Autodesk Inventor part; units mm, degrees
(part 2 of 2)
  spline S177 degree 3 poles (4.8169, 39.172) (4.6782, 38.9898) (4.5503, 38.7988) (4.3217, 38.3936) (4.2159, 38.1797) (4.0576, 37.7838) (3.993, 37.6061) (3.9199, 37.304) (3.8938, 37.1823) (3.8938, 37.0599) knots 0 0 0 0 0.294801 0.294801 0.599477 0.599477 0.842158 0.842158 1 1 1 1
  spline S178 degree 3 poles (22.2511, 37.2023) (22.2293, 37.2635) (22.2074, 37.3246) (22.1616, 37.453) (22.1204, 37.5159) (22.0066, 37.5961) (21.9396, 37.6167) (21.8732, 37.6167) knots 0 0 0 0 0.319996 0.319996 0.672558 0.672558 1 1 1 1
  spline S179 degree 2 poles (22.2511, 37.2023) (22.2677, 37.1877) (22.3899, 37.1012) (22.5179, 37.1012) knots 0.820738 0.820738 0.820738 1 2 2 2
  spline S180 degree 2 poles (22.5179, 37.1012) (22.6319, 37.1012) (22.8367, 37.2176) (22.9112, 37.3246) knots 0 0 0 1 2 2 2
  spline S181 degree 2 poles (22.9112, 37.3246) (23.0446, 37.5226) (23.0786, 38.0049) knots 0 0 0 0.924384 0.924384 0.924384
  spline S182 degree 3 poles (22.4225, 37.7192) (22.5545, 37.7192) (22.6891, 37.7457) (22.91, 37.8523) (23.001, 37.9228) (23.0786, 38.0049) knots 0 0 0 0 0.540011 0.540011 1 1 1 1
  spline S183 degree 3 poles (21.4881, 38.7257) (21.4881, 38.5944) (21.5102, 38.4625) (21.5981, 38.2196) (21.6635, 38.1074) (21.8327, 37.9218) (21.9363, 37.8474) (22.1658, 37.7449) (22.2953, 37.7192) (22.4225, 37.7192) knots 0 0 0 0 0.25832 0.25832 0.506669 0.506669 0.749947 0.749947 1 1 1 1
  spline S184 degree 3 poles (22.5505, 39.7812) (22.4044, 39.7812) (22.2546, 39.7563) (21.9944, 39.649) (21.8771, 39.5727) (21.687, 39.3809) (21.6123, 39.2629) (21.5132, 39.007) (21.4881, 38.865) (21.4881, 38.7257) knots 0 0 0 0 0.263162 0.263162 0.506642 0.506642 0.74915 0.74915 1 1 1 1
  spline S185 degree 3 poles (23.692, 38.2882) (23.692, 38.5011) (23.6719, 38.7154) (23.5699, 39.09) (23.5008, 39.2539) (23.2994, 39.5163) (23.1745, 39.617) (22.8834, 39.7517) (22.7151, 39.7812) (22.5505, 39.7812) knots 0 0 0 0 0.301479 0.301479 0.547676 0.547676 0.76686 0.76686 1 1 1 1
  spline S186 degree 3 poles (22.5016, 36.6672) (22.6714, 36.6672) (22.8436, 36.6978) (23.1467, 36.8392) (23.2768, 36.9507) (23.4893, 37.2339) (23.5642, 37.4125) (23.6719, 37.8193) (23.692, 38.0562) (23.692, 38.2882) knots 0 0 0 0 0.225089 0.225089 0.443165 0.443165 0.692425 0.692425 1 1 1 1
  spline S187 degree 3 poles (21.6021, 37.3479) (21.6021, 37.2366) (21.6487, 37.1295) (21.7902, 36.9229) (21.9024, 36.8362) (22.1707, 36.6973) (22.3382, 36.6672) (22.5016, 36.6672) knots 0 0 0 0 0.270338 0.270338 0.603095 0.603095 1 1 1 1
  spline S188 degree 3 poles (21.8732, 37.6167) (21.832, 37.6167) (21.7593, 37.6021) (21.6999, 37.5572) (21.6517, 37.5063) (21.6132, 37.447) (21.6021, 37.3773) (21.6021, 37.3479) knots 0 0 0 0 0.292922 0.512613 0.512613 0.79112 1 1 1 1
  spline S189 degree 3 poles (30.4375, 39.79) (30.4036, 39.79) (30.3434, 39.7855) (30.2892, 39.7567) (30.2556, 39.7208) (30.2301, 39.6882) (30.1801, 39.622) (30.1454, 39.5737) (30.0482, 39.4385) (29.964, 39.3461) (29.8067, 39.2089) (29.6828, 39.1259) (29.5498, 39.058) (29.4923, 39.0312) knots 0 0 0 0 0.081756 0.143072 0.143072 0.200115 0.242897 0.342722 0.342722 0.642421 0.642421 0.846752 1 1 1 1
  spline S190 degree 3 poles (30.7225, 39.4304) (30.7225, 39.5212) (30.704, 39.6157) (30.6197, 39.7246) (30.5541, 39.7767) (30.472, 39.79) (30.4375, 39.79) knots 0 0 0 0 0.529945 0.529945 0.798548 1 1 1 1
  line L67 (30.7225, 37.1263) -> (30.7225, 39.4304)
  spline S191 degree 3 poles (30.3979, 36.6714) (30.458, 36.6714) (30.5831, 36.7004) (30.6846, 36.8431) (30.7171, 36.9901) (30.7225, 37.0812) (30.7225, 37.1263) knots 0 0 0 0 0.285714 0.571429 0.785714 1 1 1 1
  spline S192 degree 3 poles (30.0756, 37.0472) (30.0756, 36.9489) (30.0968, 36.8439) (30.1964, 36.7333) (30.2718, 36.6832) (30.3606, 36.6714) (30.3979, 36.6714) knots 0 0 0 0 0.52997 0.52997 0.798558 1 1 1 1
  line L68 (30.0756, 38.7782) -> (30.0756, 37.0472)
  spline S193 degree 3 poles (29.4367, 38.4355) (29.4764, 38.4355) (29.5541, 38.4558) (29.6987, 38.5229) (29.8728, 38.6311) (30.0071, 38.7271) (30.0756, 38.7782) knots 0 0 0 0 0.162539 0.325077 0.650155 1 1 1 1
  spline S194 degree 3 poles (29.1726, 38.709) (29.1726, 38.6688) (29.1882, 38.5983) (29.2307, 38.5401) (29.2794, 38.4897) (29.337, 38.4482) (29.4071, 38.4355) (29.4367, 38.4355) knots 0 0 0 0 0.288261 0.504456 0.504456 0.787624 1 1 1 1
  spline S195 degree 3 poles (29.4923, 39.0312) (29.4457, 39.0092) (29.3647, 38.9693) (29.287, 38.9235) (29.2317, 38.8813) (29.1847, 38.8236) (29.1726, 38.75) (29.1726, 38.709) knots 0 0 0 0 0.317971 0.55645 0.55645 0.746543 1 1 1 1
  spline S196 degree 3 poles (39.388, 39.7748) (39.3541, 39.7748) (39.2939, 39.7702) (39.2397, 39.7415) (39.2101, 39.7099) (39.1842, 39.6777) (39.1341, 39.6115) (39.0958, 39.5585) (38.9987, 39.4233) (38.9145, 39.3308) (38.7572, 39.1936) (38.6333, 39.1107) (38.5003, 39.0428) (38.4428, 39.016) knots 0 0 0 0 0.081756 0.143072 0.143072 0.185854 0.242897 0.342722 0.342722 0.642421 0.642421 0.846752 1 1 1 1
  spline S197 degree 3 poles (39.673, 39.4152) (39.673, 39.506) (39.6545, 39.6005) (39.5773, 39.7002) (39.516, 39.7561) (39.434, 39.7748) (39.388, 39.7748) knots 0 0 0 0 0.529945 0.529945 0.731397 1 1 1 1
  line L69 (39.673, 37.1111) -> (39.673, 39.4152)
  spline S198 degree 3 poles (39.3484, 36.6561) (39.4085, 36.6561) (39.5335, 36.6852) (39.6351, 36.8278) (39.6676, 36.9748) (39.673, 37.066) (39.673, 37.1111) knots 0 0 0 0 0.285714 0.571429 0.785714 1 1 1 1
  spline S199 degree 3 poles (39.0261, 37.032) (39.0261, 36.9337) (39.0473, 36.8286) (39.1469, 36.7181) (39.2223, 36.668) (39.311, 36.6561) (39.3484, 36.6561) knots 0 0 0 0 0.52997 0.52997 0.798558 1 1 1 1
  line L70 (39.0261, 38.763) -> (39.0261, 37.032)
  spline S200 degree 3 poles (38.3872, 38.4203) (38.4269, 38.4203) (38.5046, 38.4406) (38.6492, 38.5077) (38.8233, 38.6159) (38.9576, 38.7119) (39.0261, 38.763) knots 0 0 0 0 0.162539 0.325077 0.650155 1 1 1 1
  spline S201 degree 3 poles (38.1231, 38.6937) (38.1231, 38.6535) (38.1387, 38.583) (38.1812, 38.5249) (38.2229, 38.4817) (38.278, 38.4376) (38.3477, 38.4203) (38.3872, 38.4203) knots 0 0 0 0 0.288261 0.504456 0.504456 0.716832 1 1 1 1
  spline S202 degree 3 poles (38.4428, 39.016) (38.3962, 38.994) (38.3152, 38.9541) (38.2375, 38.9082) (38.1822, 38.866) (38.1352, 38.8084) (38.1231, 38.7348) (38.1231, 38.6937) knots 0 0 0 0 0.317971 0.55645 0.55645 0.746543 1 1 1 1
  spline S203 degree 3 poles (48.4842, 39.7369) (48.4503, 39.7369) (48.3901, 39.7324) (48.3359, 39.7036) (48.3023, 39.6677) (48.2768, 39.6351) (48.2268, 39.569) (48.1921, 39.5207) (48.0949, 39.3854) (48.0107, 39.293) (47.8534, 39.1558) (47.7295, 39.0729) (47.5965, 39.005) (47.539, 38.9781) knots 0 0 0 0 0.081756 0.143072 0.143072 0.200115 0.242897 0.342722 0.342722 0.642421 0.642421 0.846752 1 1 1 1
  spline S204 degree 3 poles (48.7692, 39.3774) (48.7692, 39.4682) (48.7507, 39.5627) (48.6664, 39.6716) (48.6008, 39.7236) (48.5187, 39.7369) (48.4842, 39.7369) knots 0 0 0 0 0.529945 0.529945 0.798548 1 1 1 1
  line L71 (48.7692, 37.0733) -> (48.7692, 39.3774)
  spline S205 degree 3 poles (48.4446, 36.6183) (48.4897, 36.6183) (48.582, 36.6325) (48.7035, 36.7317) (48.7612, 36.8925) (48.7692, 37.0132) (48.7692, 37.0733) knots 0 0 0 0 0.214286 0.428571 0.714286 1 1 1 1
  spline S206 degree 3 poles (48.1223, 36.9942) (48.1223, 36.8959) (48.1435, 36.7908) (48.2348, 36.6896) (48.3059, 36.6349) (48.3948, 36.6183) (48.4446, 36.6183) knots 0 0 0 0 0.52997 0.52997 0.731411 1 1 1 1
  line L72 (48.1223, 38.7252) -> (48.1223, 36.9942)
  spline S207 degree 3 poles (47.4834, 38.3825) (47.5231, 38.3825) (47.6008, 38.4028) (47.7454, 38.4699) (47.9195, 38.578) (48.0538, 38.6741) (48.1223, 38.7252) knots 0 0 0 0 0.162539 0.325077 0.650155 1 1 1 1
  spline S208 degree 3 poles (47.2193, 38.6559) (47.2193, 38.6258) (47.2306, 38.5551) (47.2704, 38.4943) (47.3261, 38.4367) (47.3837, 38.3952) (47.4538, 38.3825) (47.4834, 38.3825) knots 0 0 0 0 0.216195 0.504456 0.504456 0.787624 1 1 1 1
  spline S209 degree 3 poles (47.539, 38.9781) (47.4924, 38.9562) (47.4114, 38.9162) (47.3337, 38.8704) (47.2784, 38.8282) (47.2314, 38.7706) (47.2193, 38.6969) (47.2193, 38.6559) knots 0 0 0 0 0.317971 0.55645 0.55645 0.746543 1 1 1 1
  spline S210 degree 3 poles (-13.2698, 38.7932) (-13.2836, 38.7932) (-13.2975, 38.7929) (-13.3252, 38.7915) (-13.3392, 38.7905) (-13.3602, 38.7885) (-13.3672, 38.7877) (-13.3884, 38.7852) (-13.4025, 38.7831) (-13.4238, 38.7796) (-13.4309, 38.7784) (-13.4524, 38.7743) (-13.4667, 38.7713) (-13.4882, 38.7663) (-13.4954, 38.7646) (-13.5172, 38.7591) (-13.5317, 38.7551) (-13.5534, 38.7486) (-13.5607, 38.7464) (-13.5827, 38.7394) (-13.5974, 38.7344) (-13.6194, 38.7266) (-13.6268, 38.7239) (-13.6491, 38.7154) (-13.664, 38.7095) (-13.6863, 38.7002) (-13.6937, 38.697) (-13.7019, 38.6935) (-13.7026, 38.6932) (-13.7033, 38.6929) knots 0 0 0 0 0.092703 0.092703 0.186345 0.186345 0.233583 0.233583 0.329041 0.329041 0.377326 0.377326 0.475187 0.475187 0.52484 0.52484 0.625741 0.625741 0.676923 0.676923 0.780779 0.780779 0.833489 0.833489 0.940578 0.940578 0.995003 0.995003 1 1 1 1
  spline S211 degree 3 poles (-12.2735, 37.7713) (-12.2735, 37.8182) (-12.2763, 37.8652) (-12.2863, 37.946) (-12.2922, 37.9799) (-12.3023, 38.0245) (-12.305, 38.0356) (-12.3136, 38.0685) (-12.3201, 38.0902) (-12.3308, 38.1223) (-12.3346, 38.133) (-12.3464, 38.1646) (-12.355, 38.1854) (-12.3688, 38.2159) (-12.3735, 38.226) (-12.3879, 38.2556) (-12.3981, 38.275) (-12.4144, 38.3036) (-12.4199, 38.313) (-12.4425, 38.3499) (-12.4608, 38.3768) (-12.4933, 38.4198) (-12.5069, 38.4365) (-12.5493, 38.4854) (-12.5795, 38.5159) (-12.6276, 38.5585) (-12.6439, 38.5722) (-12.6943, 38.6114) (-12.7297, 38.6354) (-12.7848, 38.6679) (-12.8036, 38.6782) (-12.8616, 38.7075) (-12.9014, 38.7248) (-12.9631, 38.7465) (-12.9841, 38.7529) (-13.0477, 38.7703) (-13.0911, 38.7789) (-13.1797, 38.7905) (-13.225, 38.7932) (-13.2698, 38.7932) knots 0 0 0 0 0.088924 0.088924 0.154115 0.154115 0.175635 0.175635 0.218439 0.218439 0.239813 0.239813 0.282415 0.282415 0.303307 0.303307 0.344643 0.344643 0.365106 0.365106 0.426005 0.426005 0.466506 0.466506 0.547908 0.547908 0.588064 0.588064 0.668181 0.668181 0.708462 0.708462 0.790774 0.790774 0.832059 0.832059 0.914902 0.914902 1 1 1 1
  spline S212 degree 3 poles (-13.4188, 36.6493) (-13.3638, 36.6493) (-13.3086, 36.6523) (-13.2013, 36.6647) (-13.1493, 36.6739) (-13.0729, 36.6928) (-13.0481, 36.6998) (-12.9871, 36.7193) (-12.9513, 36.7328) (-12.9048, 36.7533) (-12.8933, 36.7586) (-12.8592, 36.775) (-12.8369, 36.7868) (-12.8041, 36.8056) (-12.7934, 36.812) (-12.7514, 36.8379) (-12.7209, 36.8587) (-12.6724, 36.8958) (-12.6537, 36.9111) (-12.5995, 36.9588) (-12.5659, 36.9927) (-12.5191, 37.0474) (-12.5042, 37.0661) (-12.4685, 37.1143) (-12.4486, 37.1445) (-12.4241, 37.186) (-12.4182, 37.1966) (-12.4008, 37.2285) (-12.3899, 37.2501) (-12.3747, 37.2829) (-12.3698, 37.2939) (-12.351, 37.3382) (-12.3385, 37.3721) (-12.3204, 37.4297) (-12.3139, 37.453) (-12.2965, 37.524) (-12.2878, 37.5723) (-12.2763, 37.671) (-12.2735, 37.7213) (-12.2735, 37.7713) knots 0 0 0 0 0.092276 0.092276 0.180807 0.180807 0.223969 0.223969 0.287955 0.287955 0.309124 0.309124 0.351194 0.351194 0.372002 0.372002 0.43328 0.43328 0.47363 0.47363 0.553801 0.553801 0.593615 0.593615 0.653557 0.653557 0.673705 0.673705 0.713981 0.713981 0.734138 0.734138 0.794581 0.794581 0.834843 0.834843 0.916161 0.916161 1 1 1 1
  spline S213 degree 3 poles (-14.4849, 37.4571) (-14.4849, 37.4309) (-14.4824, 37.4046) (-14.4733, 37.351) (-14.4665, 37.3237) (-14.4537, 37.2829) (-14.4488, 37.2689) (-14.4352, 37.2331) (-14.426, 37.2115) (-14.4126, 37.1829) (-14.4091, 37.1755) (-14.3999, 37.1569) (-14.3941, 37.1458) (-14.3861, 37.1308) (-14.3841, 37.1269) (-14.3776, 37.1151) (-14.373, 37.1072) (-14.3659, 37.0954) (-14.3635, 37.0914) (-14.3535, 37.0757) (-14.3457, 37.0641) (-14.332, 37.0451) (-14.3263, 37.0376) (-14.3087, 37.015) (-14.2963, 37.0004) (-14.2768, 36.9789) (-14.2701, 36.9718) (-14.2421, 36.9432) (-14.2199, 36.9227) (-14.1809, 36.89) (-14.1645, 36.8771) (-14.1258, 36.8484) (-14.1034, 36.833) (-14.0759, 36.8153) (-14.0711, 36.8123) (-14.0568, 36.8033) (-14.0471, 36.7974) (-14.0322, 36.7887) (-14.0271, 36.7857) (-14.0062, 36.774) (-13.9901, 36.7656) (-13.9629, 36.7525) (-13.9518, 36.7475) (-13.9061, 36.7277) (-13.8707, 36.715) (-13.8099, 36.6966) (-13.7847, 36.69) (-13.7059, 36.6721) (-13.6514, 36.6636) (-13.5374, 36.6519) (-13.4778, 36.6493) (-13.4188, 36.6493) knots 0 0 0 0 0.05342 0.05342 0.110323 0.110323 0.140525 0.140525 0.188212 0.188212 0.204851 0.204851 0.230452 0.230452 0.239326 0.239326 0.257866 0.257866 0.26723 0.26723 0.295467 0.295467 0.314492 0.314492 0.353157 0.353157 0.372878 0.372878 0.434045 0.434045 0.476554 0.476554 0.531612 0.531612 0.542912 0.542912 0.565933 0.565933 0.577878 0.577878 0.614515 0.614515 0.639286 0.639286 0.715798 0.715798 0.768641 0.768641 0.879679 0.879679 1 1 1 1
  spline S214 degree 3 poles (-14.1845, 37.7482) (-14.198, 37.7482) (-14.2116, 37.7474) (-14.2384, 37.744) (-14.2515, 37.7414) (-14.2709, 37.7361) (-14.2773, 37.7342) (-14.2962, 37.7276) (-14.3084, 37.7223) (-14.3261, 37.7131) (-14.3319, 37.7098) (-14.3461, 37.701) (-14.3543, 37.6953) (-14.365, 37.6871) (-14.3676, 37.685) (-14.3754, 37.6786) (-14.3804, 37.6741) (-14.3878, 37.6672) (-14.3902, 37.6648) (-14.3973, 37.6576) (-14.4019, 37.6527) (-14.4084, 37.6454) (-14.4105, 37.643) (-14.4166, 37.6358) (-14.4206, 37.6309) (-14.4264, 37.6233) (-14.4282, 37.6208) (-14.4355, 37.6107) (-14.4407, 37.603) (-14.4486, 37.5897) (-14.4516, 37.5844) (-14.46, 37.5682) (-14.465, 37.5571) (-14.4712, 37.54) (-14.4731, 37.5342) (-14.4781, 37.5169) (-14.4807, 37.505) (-14.4841, 37.4812) (-14.4849, 37.4691) (-14.4849, 37.4571) knots 0 0 0 0 0.088245 0.088245 0.175465 0.175465 0.21879 0.21879 0.305396 0.305396 0.348669 0.348669 0.41348 0.41348 0.435158 0.435158 0.478569 0.478569 0.5006 0.5006 0.543973 0.543973 0.564583 0.564583 0.605632 0.605632 0.625924 0.625924 0.68612 0.68612 0.725881 0.725881 0.804934 0.804934 0.844081 0.844081 0.921896 0.921896 1 1 1 1
  spline S215 degree 3 poles (-13.8701, 37.5135) (-13.88, 37.5366) (-13.8912, 37.5593) (-13.9133, 37.5962) (-13.9234, 37.611) (-13.9381, 37.6297) (-13.9418, 37.6342) (-13.9531, 37.6473) (-13.961, 37.6557) (-13.9734, 37.6675) (-13.9777, 37.6713) (-13.9905, 37.6823) (-13.9995, 37.6892) (-14.0135, 37.6988) (-14.0182, 37.7019) (-14.0326, 37.7106) (-14.0425, 37.7158) (-14.0578, 37.7228) (-14.0629, 37.725) (-14.0785, 37.7311) (-14.0892, 37.7346) (-14.1055, 37.739) (-14.111, 37.7403) (-14.1276, 37.7437) (-14.1388, 37.7454) (-14.1616, 37.7477) (-14.1731, 37.7482) (-14.1845, 37.7482) knots 0 0 0 0 0.180992 0.180992 0.309668 0.309668 0.351501 0.351501 0.434189 0.434189 0.475017 0.475017 0.555697 0.555697 0.595796 0.595796 0.676019 0.676019 0.716301 0.716301 0.796698 0.796698 0.836889 0.836889 0.917728 0.917728 1 1 1 1
  ellipse E0 centre (-13.6776, 37.5949) end of major axis (-13.766, 37.7956) minor radius 0.2091 (-13.8701, 37.5135) -> (-13.8672, 37.5069) ccw
  spline S216 degree 3 poles (-13.4095, 37.1734) (-13.4255, 37.1734) (-13.4416, 37.1741) (-13.4732, 37.1773) (-13.4887, 37.1797) (-13.5114, 37.1844) (-13.5189, 37.1862) (-13.5411, 37.1921) (-13.5556, 37.1968) (-13.5769, 37.205) (-13.5839, 37.2079) (-13.605, 37.2174) (-13.6188, 37.2245) (-13.6391, 37.2363) (-13.6458, 37.2405) (-13.6661, 37.2537) (-13.6792, 37.2634) (-13.6984, 37.2788) (-13.7047, 37.2841) (-13.7235, 37.3007) (-13.7355, 37.3123) (-13.7528, 37.3307) (-13.7586, 37.3371) (-13.7755, 37.3568) (-13.7864, 37.3706) (-13.8019, 37.3921) (-13.807, 37.3995) (-13.8222, 37.4225) (-13.8318, 37.4385) (-13.8503, 37.4719) (-13.8591, 37.4893) (-13.8672, 37.5069) knots 0 0 0 0 0.080666 0.080666 0.158277 0.158277 0.196485 0.196485 0.272757 0.272757 0.311136 0.311136 0.388673 0.388673 0.428088 0.428088 0.509412 0.509412 0.550797 0.550797 0.634906 0.634906 0.677634 0.677634 0.764932 0.764932 0.809746 0.809746 0.902371 0.902371 1 1 1 1
  spline S217 degree 3 poles (-12.9651, 37.7248) (-12.9651, 37.6979) (-12.9663, 37.6709) (-12.9711, 37.6187) (-12.9746, 37.5935) (-12.9819, 37.5567) (-12.9845, 37.5448) (-12.9933, 37.51) (-13.0004, 37.4874) (-13.0128, 37.4544) (-13.0172, 37.4438) (-13.0309, 37.4131) (-13.041, 37.3935) (-13.0581, 37.3655) (-13.0639, 37.3566) (-13.0818, 37.3312) (-13.0948, 37.3153) (-13.1157, 37.293) (-13.1229, 37.286) (-13.1451, 37.2655) (-13.161, 37.2529) (-13.186, 37.2359) (-13.1945, 37.2305) (-13.2203, 37.2156) (-13.2382, 37.2071) (-13.2658, 37.1966) (-13.2752, 37.1934) (-13.3043, 37.1848) (-13.3243, 37.1805) (-13.3661, 37.1747) (-13.3879, 37.1734) (-13.4095, 37.1734) knots 0 0 0 0 0.101982 0.101982 0.198078 0.198078 0.244289 0.244289 0.333652 0.333652 0.37732 0.37732 0.460741 0.460741 0.500448 0.500448 0.577702 0.577702 0.615856 0.615856 0.691855 0.691855 0.729606 0.729606 0.804116 0.804116 0.841589 0.841589 0.918244 0.918244 1 1 1 1
  spline S218 degree 3 poles (-13.4025, 38.2576) (-13.3823, 38.2576) (-13.362, 38.2564) (-13.3228, 38.2515) (-13.3039, 38.2479) (-13.2763, 38.2406) (-13.2673, 38.2379) (-13.2407, 38.2289) (-13.2235, 38.2217) (-13.1985, 38.2091) (-13.1902, 38.2047) (-13.1663, 38.1905) (-13.1511, 38.1798) (-13.1297, 38.162) (-13.1227, 38.1558) (-13.1019, 38.1357) (-13.089, 38.1212) (-13.0708, 38.0976) (-13.0649, 38.0892) (-13.0471, 38.0626) (-13.0362, 38.0436) (-13.0214, 38.0139) (-13.0167, 38.0036) (-13.0032, 37.9713) (-12.9957, 37.949) (-12.9862, 37.9141) (-12.9834, 37.902) (-12.9754, 37.8639) (-12.9716, 37.8376) (-12.9663, 37.7824) (-12.9651, 37.7534) (-12.9651, 37.7248) knots 0 0 0 0 0.07838 0.07838 0.152885 0.152885 0.18919 0.18919 0.261457 0.261457 0.297443 0.297443 0.36848 0.36848 0.404641 0.404641 0.480054 0.480054 0.519572 0.519572 0.603431 0.603431 0.647357 0.647357 0.738828 0.738828 0.786932 0.786932 0.888762 0.888762 1 1 1 1
  spline S219 degree 3 poles (-14.0937, 37.962) (-14.0827, 37.962) (-14.0717, 37.9628) (-14.0497, 37.9658) (-14.0387, 37.968) (-14.0223, 37.9722) (-14.0168, 37.9738) (-13.9942, 37.9809) (-13.9777, 37.9874) (-13.95, 38.0001) (-13.9387, 38.0058) (-13.9098, 38.0216) (-13.8924, 38.0323) (-13.8694, 38.0474) (-13.8634, 38.0515) (-13.8483, 38.062) (-13.8392, 38.0685) (-13.8272, 38.0775) (-13.8241, 38.0797) (-13.8154, 38.0863) (-13.8097, 38.0906) (-13.8013, 38.097) (-13.7985, 38.099) (-13.7878, 38.1071) (-13.7797, 38.1131) (-13.7666, 38.1228) (-13.7615, 38.1265) (-13.7467, 38.1373) (-13.7369, 38.1443) (-13.7226, 38.1545) (-13.718, 38.1577) (-13.7048, 38.167) (-13.6962, 38.1729) (-13.6835, 38.1816) (-13.6794, 38.1843) (-13.6679, 38.1919) (-13.6604, 38.1969) (-13.6494, 38.2039) (-13.6459, 38.2061) (-13.6376, 38.2112) (-13.6328, 38.2142) (-13.6265, 38.218) (-13.625, 38.2189) (-13.6213, 38.221) (-13.6191, 38.2223) (-13.6163, 38.2239) (-13.6156, 38.2242) (-13.614, 38.2251) (-13.613, 38.2257) (-13.6115, 38.2265) (-13.6109, 38.2268) (-13.6076, 38.2284) (-13.6047, 38.2298) (-13.5991, 38.2321) (-13.5964, 38.2332) (-13.5839, 38.2378) (-13.5737, 38.2406) (-13.5553, 38.245) (-13.5469, 38.2466) (-13.5185, 38.2515) (-13.4981, 38.2537) (-13.4525, 38.2569) (-13.4273, 38.2576) (-13.4025, 38.2576) knots 0 0 0 0 0.042878 0.042878 0.086235 0.086235 0.108331 0.108331 0.177769 0.177769 0.226997 0.226997 0.306227 0.306227 0.334276 0.334276 0.378117 0.378117 0.392867 0.392867 0.420693 0.420693 0.434144 0.434144 0.473134 0.473134 0.49792 0.49792 0.54464 0.54464 0.56656 0.56656 0.607505 0.607505 0.62651 0.62651 0.661461 0.661461 0.677346 0.677346 0.699322 0.699322 0.706098 0.706098 0.715907 0.715907 0.718762 0.718762 0.723223 0.723223 0.725491 0.725491 0.737857 0.737857 0.749199 0.749199 0.790187 0.790187 0.823398 0.823398 0.902976 0.902976 1 1 1 1
  spline S220 degree 3 poles (-14.4151, 38.269) (-14.4151, 38.2676) (-14.4151, 38.2661) (-14.4151, 38.2514) (-14.4141, 38.2381) (-14.4103, 38.2117) (-14.4074, 38.1987) (-14.4016, 38.1797) (-14.3994, 38.1734) (-14.3922, 38.1547) (-14.3864, 38.1427) (-14.3766, 38.1253) (-14.3731, 38.1195) (-14.3619, 38.1026) (-14.3537, 38.0918) (-14.3403, 38.0763) (-14.3356, 38.0712) (-14.321, 38.0562) (-14.3108, 38.0467) (-14.2946, 38.0333) (-14.2891, 38.029) (-14.2725, 38.0168) (-14.261, 38.0093) (-14.2432, 37.9992) (-14.2372, 37.9961) (-14.219, 37.9872) (-14.2065, 37.9821) (-14.1872, 37.9757) (-14.1807, 37.9738) (-14.1611, 37.9687) (-14.1478, 37.9662) (-14.1209, 37.9628) (-14.1072, 37.962) (-14.0937, 37.962) knots 0 0 0 0 0.008781 0.008781 0.090256 0.090256 0.170943 0.170943 0.211408 0.211408 0.29299 0.29299 0.333922 0.333922 0.416357 0.416357 0.458304 0.458304 0.544271 0.544271 0.586412 0.586412 0.669662 0.669662 0.711114 0.711114 0.793793 0.793793 0.834866 0.834866 0.916953 0.916953 1 1 1 1
  line L73 (-14.2222, 39.3838) -> (-14.4151, 38.269)
  spline S221 degree 3 poles (-13.8005, 39.7661) (-13.8204, 39.7661) (-13.8405, 39.7653) (-13.8792, 39.7622) (-13.8979, 39.7598) (-13.9253, 39.7548) (-13.9341, 39.7529) (-13.9598, 39.7467) (-13.9765, 39.7416) (-14.0007, 39.7323) (-14.0085, 39.729) (-14.0275, 39.72) (-14.0385, 39.714) (-14.0526, 39.7052) (-14.0561, 39.7029) (-14.0663, 39.6959) (-14.0728, 39.6909) (-14.0823, 39.6831) (-14.0855, 39.6804) (-14.0974, 39.6696) (-14.1058, 39.6609) (-14.1188, 39.6457) (-14.1237, 39.6396) (-14.1381, 39.6202) (-14.1469, 39.6065) (-14.1589, 39.5851) (-14.1627, 39.5777) (-14.174, 39.5547) (-14.1807, 39.5387) (-14.1898, 39.514) (-14.1927, 39.5055) (-14.2012, 39.479) (-14.2061, 39.4608) (-14.215, 39.4231) (-14.2189, 39.4035) (-14.2222, 39.3838) knots 0 0 0 0 0.094223 0.094223 0.182563 0.182563 0.225056 0.225056 0.307372 0.307372 0.347176 0.347176 0.405824 0.405824 0.425239 0.425239 0.463974 0.463974 0.483411 0.483411 0.540187 0.540187 0.577263 0.577263 0.653772 0.653772 0.693184 0.693184 0.774599 0.774599 0.816883 0.816883 0.905528 0.905528 1 1 1 1
  line L74 (-12.7392, 39.7661) -> (-13.8005, 39.7661)
  spline S222 degree 3 poles (-12.355, 39.4563) (-12.355, 39.4719) (-12.3558, 39.4875) (-12.3594, 39.5179) (-12.3622, 39.5327) (-12.3679, 39.5545) (-12.37, 39.5616) (-12.3772, 39.5826) (-12.3831, 39.5961) (-12.3936, 39.6154) (-12.3973, 39.6218) (-12.4093, 39.6401) (-12.4184, 39.6517) (-12.4334, 39.6677) (-12.4387, 39.6728) (-12.455, 39.6876) (-12.4668, 39.6965) (-12.4854, 39.7085) (-12.4919, 39.7123) (-12.5117, 39.7232) (-12.5256, 39.7294) (-12.5469, 39.7376) (-12.5543, 39.7401) (-12.5769, 39.7472) (-12.5924, 39.7511) (-12.6162, 39.7559) (-12.6244, 39.7573) (-12.6497, 39.7612) (-12.6669, 39.763) (-12.7025, 39.7655) (-12.7209, 39.7661) (-12.7392, 39.7661) knots 0 0 0 0 0.083384 0.083384 0.164256 0.164256 0.203964 0.203964 0.282774 0.282774 0.321879 0.321879 0.399682 0.399682 0.4388 0.4388 0.517693 0.517693 0.557347 0.557347 0.638 0.638 0.679552 0.679552 0.765316 0.765316 0.809642 0.809642 0.901852 0.901852 1 1 1 1
  spline S223 degree 3 poles (-12.7275, 39.1536) (-12.7099, 39.1536) (-12.6921, 39.1542) (-12.6577, 39.1569) (-12.641, 39.1589) (-12.6165, 39.1631) (-12.6085, 39.1646) (-12.5853, 39.1699) (-12.5701, 39.1741) (-12.548, 39.1818) (-12.5408, 39.1846) (-12.5233, 39.192) (-12.5131, 39.1969) (-12.4998, 39.2042) (-12.4966, 39.2061) (-12.487, 39.2119) (-12.4807, 39.2159) (-12.4716, 39.2224) (-12.4686, 39.2246) (-12.4599, 39.2313) (-12.4543, 39.236) (-12.4462, 39.2432) (-12.4436, 39.2456) (-12.436, 39.2529) (-12.4311, 39.2579) (-12.424, 39.2657) (-12.4217, 39.2684) (-12.4128, 39.2791) (-12.4065, 39.2875) (-12.3968, 39.3021) (-12.3932, 39.308) (-12.3831, 39.3264) (-12.3773, 39.3391) (-12.3702, 39.3587) (-12.368, 39.3654) (-12.3623, 39.3856) (-12.3595, 39.3995) (-12.3558, 39.4277) (-12.355, 39.4421) (-12.355, 39.4563) knots 0 0 0 0 0.098484 0.098484 0.191898 0.191898 0.236946 0.236946 0.324302 0.324302 0.367026 0.367026 0.429927 0.429927 0.450621 0.450621 0.491663 0.491663 0.512232 0.512232 0.55254 0.55254 0.572021 0.572021 0.611128 0.611128 0.630547 0.630547 0.688397 0.688397 0.726878 0.726878 0.804248 0.804248 0.843006 0.843006 0.920729 0.920729 1 1 1 1
  line L75 (-13.6229, 39.1536) -> (-12.7275, 39.1536)
  line L76 (-13.7033, 38.6929) -> (-13.6229, 39.1536)
  line L77 (13.8521, 32) -> (13.8521, -32)
  line L78 (13.8521, -32) -> (-12.1479, -32)
  line L79 (-12.1479, -32) -> (-12.1479, 32)
  line L80 (-12.1479, 32) -> (13.8521, 32)
  line L81 (13.8521, 32) -> (-12.1479, -32) construction
  line L82 (13.8521, -32) -> (-12.1479, 32) construction
  line L83 (13.8521, 32) -> (77.8521, 32) construction
  point P0 (0.8521, 0)
  dimension "d2" = 64
  dimension "d3" = 90
  dimension "d4" = 26
  constraints: 14 end point, 2 midpoint, 2 parallel, 2 perpendicular, 1 horizontal, 1 vertical, 1 other
  measures "d2" distance of L77.start L77.end
  measures "d3" angle of L77 L83
  measures "d4" distance of L77.end L78.end
extrude "Extrusion2" cut sketch "Sketch2" against normal through all contours L77 L78 L79 L80
sketch "Sketch3" plane through (-0.8521, 0, -9) normal (0, 0, 1) x (1, 0, 0)
  line L0 (-12.1479, 32) -> (13.8521, 32) projected
  line L1 (13.8521, 32) -> (13.8521, -32) projected
  line L2 (13.8521, -32) -> (-12.1479, -32) projected
  line L3 (-12.1479, -32) -> (-12.1479, 32) projected
  line L4 (59.9, 42.7) -> (-59.9, 42.7) projected
  arc A0 (-59.9, 42.7) -> (-63.8, 38.8) centre (-59.9, 38.8) ccw projected
  line L5 (-63.8, 38.8) -> (-63.8, -38.8) projected
  arc A1 (-63.8, -38.8) -> (-59.9, -42.7) centre (-59.9, -38.8) ccw projected
  line L6 (-59.9, -42.7) -> (59.9, -42.7) projected
  arc A2 (59.9, -42.7) -> (63.8, -38.8) centre (59.9, -38.8) ccw projected
  line L7 (63.8, -38.8) -> (63.8, 38.8) projected
  arc A3 (63.8, 38.8) -> (59.9, 42.7) centre (59.9, 38.8) ccw projected
  line L8 (13.8521, 38) -> (13.8521, -38)
  line L9 (13.8521, -38) -> (-12.1479, -38)
  line L10 (-12.1479, -38) -> (-12.1479, 38)
  line L11 (-12.1479, 38) -> (13.8521, 38)
  line L12 (13.8521, 38) -> (-12.1479, -38) construction
  line L13 (13.8521, -38) -> (-12.1479, 38) construction
  line L14 (13.8521, 38) -> (89.8521, 38) construction
  point P0 (0.8521, 0)
  dimension "d7" = 76
  dimension "d8" = 90
  dimension "d9" = 26
  constraints: 14 end point, 2 midpoint, 2 parallel, 2 perpendicular, 1 horizontal, 1 vertical
  measures "d7" distance of L8.start L8.end
  measures "d8" angle of L8 L14
  measures "d9" distance of L8.end L9.end
extrude "Extrusion3" cut sketch "Sketch3" against normal blind 2.5 contours L10 L11 L8 L0 | L2 L8 L9 L10
pattern_linear "Rectangular Pattern1" count 3 spacing 30 along (-1, 0, 0) of "Extrusion2", "Extrusion3" first direction both ways yes
body "Solid1"
